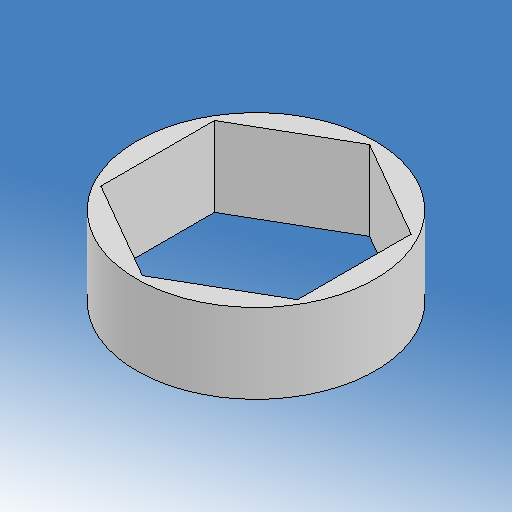
# Autodesk Inventor part: SportGearbox_HexDiffGearSpacer
Saved by Autodesk Inventor 2025 (Build 290162000, 162)
## iProperties
Created: 2024-04-23
Part Number: SportGearbox_HexDiffGearSpacer
Material: Generic
Document SubType Name: Modeling
Designer: seene
Density: 1 g/cm^3
Appearance: Default
Author: seene
Autodesk Inventor part; units mm, degrees
ref_plane "YZ Plane" through (0, 0, 0) normal (1, 0, 0) x (0, 1, 0)
ref_plane "XZ Plane" through (0, 0, 0) normal (0, 1, 0) x (-1, 0, 0)
ref_plane "XY Plane" through (0, 0, 0) normal (0, 0, 1) x (1, 0, 0)
sketch "Sketch1" plane through (0, 0, 0) normal (0, 1, 0) x (-1, 0, 0)
  circle A0 centre (0, 0) radius 6.35 construction
  line L0 (6.35, -3.6662) -> (0, -7.3323)
  line L1 (0, -7.3323) -> (-6.35, -3.6662)
  line L2 (-6.35, -3.6662) -> (-6.35, 3.6662)
  line L3 (-6.35, 3.6662) -> (0, 7.3323)
  line L4 (0, 7.3323) -> (6.35, 3.6662)
  line L5 (6.35, 3.6662) -> (6.35, -3.6662)
  circle A1 centre (0, 0) radius 9.525
  point P0 (6.35, 0)
  dimension "d0" = 12.7
  dimension "d1" = 19.05
  constraints: 12 end point, 3 coincident, 1 centre point, 1 horizontal alignment, 1 midpoint, 15 other
  measures "d1" diameter of A1
extrude "Extrusion1" add sketch "Sketch1" along normal blind 6.35
sketch "Sketch2" plane through (0, 6.35, 0) normal (0, 1, 0) x (1, 0, 0)
  line L0 (-6.35, 3.6662) -> (0, 7.3323) projected
  line L1 (0, 7.3323) -> (6.35, 3.6662) projected
  line L2 (-6.35, -3.6662) -> (-6.35, 3.6662) projected
  line L3 (0, -7.3323) -> (-6.35, -3.6662) projected
  line L4 (6.35, -3.6662) -> (0, -7.3323) projected
  line L5 (6.35, 3.6662) -> (6.35, -3.6662) projected
  line L6 (-7.85, 4.5322) -> (0, 9.0644)
  line L7 (0, 9.0644) -> (7.85, 4.5322)
  line L8 (7.85, 4.5322) -> (7.85, -4.5322)
  line L9 (7.85, -4.5322) -> (0, -9.0644)
  line L10 (0, -9.0644) -> (-7.85, -4.5322)
  line L11 (-7.85, -4.5322) -> (-7.85, 4.5322)
  point P0 (0, 0)
  dimension "d4" = 1.5
  constraints: 12 end point, 5 other
  measures "d4" distance between parallel lines of L2 L11
extrude "Extrusion2" cut sketch "Sketch2" against normal blind 25.4 contours L0 L1 L5 L4 L3 L2 | L6 L7 L8 L9 L10 L11
body "Solid1"
